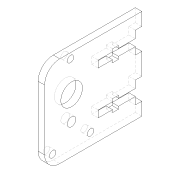
# Autodesk Inventor part: motor mount
Saved by Autodesk Inventor 2016 (Build 200138000, 138)
## iProperties
Created: 2014-07-12
Part Number: motor mount
Material: Plywood, Finish
Document SubType Name: Modeling
Designer: Sebastian
Density: 0.552 g/cm^3
Appearance: Plywood - New
Description: http://www.wickes.co.uk/Wickes-Non-Structural-Hardwood-Plywood-3-6x607x1829mm/p/110513
Mass: 2.60551 g
Surface Area: 41.387 cm^2
Volume: 4.72013 cm^3
Author: Sebastian
Autodesk Inventor part; units mm, degrees
ref_plane "YZ Plane" through (0, 0, 0) normal (1, 0, 0) x (0, 1, 0)
ref_plane "XZ Plane" through (0, 0, 0) normal (0, 1, 0) x (-1, 0, 0)
ref_plane "XY Plane" through (0, 0, 0) normal (0, 0, 1) x (1, 0, 0)
sketch "Sketch1" plane through (0, 0, 0) normal (1, 0, 0) x (0, 1, 0)
  line L0 (0, 0) -> (45, 0)
  line L1 (45, 0) -> (45, -42)
  line L2 (45, -42) -> (0, -42)
  line L3 (0, -42) -> (0, 0)
  dimension "d0" = 45
  dimension "d1" = 42
  constraints: 8 end point, 2 parallel, 1 horizontal, 1 perpendicular
  measures "d0" distance of L1.end L2.end
  measures "d1" distance of L0.end L1.end
extrude "Extrusion1" add sketch "Sketch1" along normal blind 3
sketch "Sketch4" plane through (0, 0, 0) normal (-1, 0, 0) x (0, 0, 1)
  circle A0 centre (-2.5714, 12) radius 1.5
  circle A1 centre (-36.5714, 21.25) radius 1.5
  circle A2 centre (-36.5714, 3.75) radius 1.5
  circle A3 centre (-16.9627, 12.5) radius 5
  line L0 (-42, 0) -> (0, 0) projected
  circle A4 centre (-27.9627, 12.5) radius 2
  point P0 (0, 10)
  point P1 (-32, 0)
  point P2 (-10, 0)
  dimension "d21" = 3
  dimension "d23" = 3
  dimension "d26" = 3
  dimension "d29" = 10
  dimension "d32" = 12.5
  dimension "d76" = 4
  dimension "d77" = 4
  dimension "d78" = 12.5
  dimension "d79" = 7.9
  constraints: 5 centre point
  measures "d21" diameter of A0
  measures "d23" diameter of A1
  measures "d26" diameter of A2
  measures "d29" diameter of A3
  measures "d32" distance from line of L0 A3.centre
  measures "d76" diameter of A4
  measures "d78" distance from line of A4.centre L0
extrude "Extrusion4" cut sketch "Sketch4" against normal blind 4
sketch "Sketch5" plane through (0, 0, 0) normal (-1, 0, 0) x (0, 0, 1)
  line L0 (-16, 45) -> (-16, 42)
  line L1 (-26, 42) -> (-26, 45)
  line L2 (-36, 45) -> (-36, 42)
  line L3 (-42, 42) -> (-42, 45)
  line L4 (-6, 45) -> (-6, 42)
  line L5 (-42, 45) -> (0, 45) projected
  line L6 (-6, 45) -> (-16, 45)
  line L7 (-16, 42) -> (-16, 45)
  line L8 (-26, 45) -> (-36, 45)
  line L9 (-9.4, 24.8) -> (-12.6, 24.8)
  line L10 (-9.4, 34.2) -> (-8.2, 34.2)
  line L11 (-8.2, 34.2) -> (-8.2, 31.45)
  line L12 (-8.2, 31.45) -> (-9.4, 31.45)
  line L13 (-12.6, 34.2) -> (-13.8, 34.2)
  line L14 (-13.8, 34.2) -> (-13.8, 31.45)
  line L15 (-12.6, 31.45) -> (-13.8, 31.45)
  line L16 (-9.4, 42) -> (-9.4, 34.2)
  line L17 (-9.4, 31.45) -> (-9.4, 24.8)
  line L18 (-12.6, 24.8) -> (-12.6, 31.45)
  line L19 (-12.6, 34.2) -> (-12.6, 42)
  line L20 (-6, 42) -> (-9.4, 42)
  line L21 (-12.6, 42) -> (-16, 42)
  line L22 (-26, 42) -> (-29.4, 42)
  line L23 (-29.4, 42) -> (-29.4, 34.2)
  line L24 (-29.4, 34.2) -> (-28.2, 34.2)
  line L25 (-28.2, 34.2) -> (-28.2, 31.45)
  line L26 (-28.2, 31.45) -> (-29.4, 31.45)
  line L27 (-29.4, 31.45) -> (-29.4, 24.8)
  line L28 (-29.4, 24.8) -> (-32.6, 24.8)
  line L29 (-32.6, 24.8) -> (-32.6, 31.45)
  line L30 (-32.6, 31.45) -> (-33.8, 31.45)
  line L31 (-33.8, 31.45) -> (-33.8, 34.2)
  line L32 (-33.8, 34.2) -> (-32.6, 34.2)
  line L33 (-32.6, 34.2) -> (-32.6, 42)
  line L34 (-32.6, 42) -> (-36, 42)
  dimension "d38" = 10
  dimension "d42" = 6
  dimension "d47" = 10
  dimension "d48" = 10
  dimension "d55" = 2.75
  dimension "d59" = 3
  dimension "d60" = 7.8
  dimension "d61" = 6.65
  dimension "d62" = 5.6
  dimension "d63" = 3.2
  dimension "d64" = 3.4
  dimension "d65" = 3.4
  dimension "d66" = 7.8
  dimension "d67" = 1.2
  dimension "d68" = 1.2
  dimension "d69" = 2.75
  dimension "d70" = 3.2
  dimension "d71" = 1.2
  dimension "d72" = 1.2
  dimension "d73" = 6.65
  dimension "d74" = 7.8
  dimension "d75" = 20.2
  constraints: 68 end point, 10 perpendicular, 6 horizontal, 5 point on line, 2 collinear, 2 parallel, 1 vertical
  measures "d38" distance of L0.end L1.start
  measures "d42" distance of L2.end L3.start
  measures "d47" distance between parallel lines of L4 L0
  measures "d48" distance between parallel lines of L2 L1
  measures "d55" distance from line of L11.end L10
  measures "d59" distance of L4.start L4.end
  measures "d60" distance of L16.start L10.start
  measures "d61" distance of L12.end L9.start
  measures "d62" distance between parallel lines of L14 L11
  measures "d63" distance between parallel lines of L18 L17
  measures "d64" distance between parallel lines of L16 L4
  measures "d65" distance of L1.start L22.end
  measures "d66" distance of L22.end L23.end
  measures "d67" distance between parallel lines of L19 L14
  measures "d68" distance of L23.end L24.end
  measures "d69" distance of L24.end L25.end
  measures "d70" distance of L27.end L28.end
  measures "d71" distance of L29.end L30.end
  measures "d72" distance of L31.end L32.end
  measures "d73" distance between parallel lines of L28 L26
  measures "d74" distance between parallel lines of L24 L22
  measures "d75" distance between parallel lines of L9 L5
extrude "Extrusion5" cut sketch "Sketch5" against normal blind 4
fillet "Fillet2" radius 7 2 edges at (1.5, 0, 0) (1.5, 0, -42)
body "Solid1"
